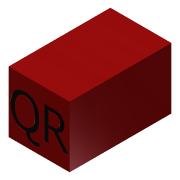
# Autodesk Inventor part: Container 2 2 2 and half color 4
Saved by Autodesk Inventor 2015 (Build 190159000, 159)
## iProperties
Created: 2015-03-07
Part Number: Container 2 2 2 and half color 4
Material: Generic
Document SubType Name: Modeling
Designer: Vukica
Density: 1 g/cm^3
Appearance: Red
Author: Vukica
Autodesk Inventor part; units mm, degrees
ref_plane "YZ Plane" through (0, 0, 0) normal (1, 0, 0) x (0, 1, 0)
ref_plane "XZ Plane" through (0, 0, 0) normal (0, 1, 0) x (-1, 0, 0)
ref_plane "XY Plane" through (0, 0, 0) normal (0, 0, 1) x (1, 0, 0)
sketch "Sketch1" plane through (0, 0, 0) normal (0, 0, 1) x (1, 0, 0)
  line L0 (0, 0) -> (38.1, 0)
  line L1 (38.1, 0) -> (38.1, 38.1)
  line L2 (38.1, 38.1) -> (0, 38.1)
  line L3 (0, 38.1) -> (0, 0)
  dimension "d0" = 38.1
  dimension "d1" = 38.1
  constraints: 8 end point, 2 parallel, 1 horizontal, 1 perpendicular
  measures "d0" distance of L1.end L2.end
  measures "d1" distance of L2.end L0.start
extrude "Extrusion1" add sketch "Sketch1" along normal blind 63.5
sketch "Sketch2" plane through (0, 0, 63.5) normal (0, 0, 1) x (1, 0, 0)
  line L0 (0.2209, 29.4428) -> (23.4184, 29.4428) construction
  line L1 (23.4184, 29.4428) -> (23.4184, 13.1304) construction
  line L2 (23.4184, 13.1304) -> (0.2209, 13.1304) construction
  line L3 (0.2209, 13.1304) -> (0.2209, 29.4428) construction
  spline S0 degree 2 poles (19.1577, 3.7217) (18.4167, 3.5406) (16.8029, 3.343) (15.996, 3.343) knots 0 0 0 1 2 2 2
  spline S1 degree 2 poles (15.996, 3.343) (13.7072, 3.343) (10.8584, 5.8953) (10.7267, 8.2666) knots 0 0 0 1 2 2 2
  spline S2 degree 2 poles (10.7267, 8.2666) (10.5455, 8.2666) (10.2327, 8.2666) (10.1009, 8.2666) knots 0 0 0 1 2 2 2
  spline S3 degree 2 poles (10.1009, 8.2666) (8.0426, 8.2666) (4.7328, 9.6662) (3.5472, 11.033) knots 0 0 0 1 2 2 2
  spline S4 degree 2 poles (3.5472, 11.033) (2.378, 12.3833) (1.1265, 16.3353) (1.1265, 18.8382) knots 0 0 0 1 2 2 2
  spline S5 degree 2 poles (1.1265, 18.8382) (1.1265, 21.407) (2.3945, 25.2932) (3.5636, 26.6764) knots 0 0 0 1 2 2 2
  spline S6 degree 2 poles (3.5636, 26.6764) (4.7492, 28.0432) (8.0591, 29.4428) (10.1009, 29.4428) knots 0 0 0 1 2 2 2
  spline S7 degree 2 poles (10.1009, 29.4428) (12.1758, 29.4428) (15.502, 27.9938) (16.6547, 26.6764) knots 0 0 0 1 2 2 2
  spline S8 degree 2 poles (16.6547, 26.6764) (17.8074, 25.3426) (19.0918, 21.3741) (19.0918, 18.8382) knots 0 0 0 1 2 2 2
  spline S9 degree 2 poles (19.0918, 18.8382) (19.0918, 14.8862) (16.0125, 9.7486) (13.3284, 8.8429) knots 0 0 0 1 2 2 2
  spline S10 degree 2 poles (13.3284, 8.8429) (13.3943, 8.0854) (13.7895, 6.8669) (14.1024, 6.5211) knots 0 0 0 1 2 2 2
  spline S11 degree 2 poles (14.1024, 6.5211) (14.4811, 6.0929) (15.5185, 5.6977) (16.4406, 5.6977) knots 0 0 0 1 2 2 2
  spline S12 degree 2 poles (16.4406, 5.6977) (16.9841, 5.6977) (18.4661, 6.0435) (18.7954, 6.1753) knots 0 0 0 1 2 2 2
  line L4 (18.7954, 6.1753) -> (19.1577, 6.1753)
  line L5 (19.1577, 6.1753) -> (19.1577, 3.7217)
  spline S13 degree 2 poles (16.276, 18.8382) (16.276, 20.8636) (15.4032, 23.9759) (14.6128, 24.9968) knots 0 0 0 1 2 2 2
  spline S14 degree 2 poles (14.6128, 24.9968) (13.806, 26.0507) (11.5335, 27.1045) (10.1174, 27.1045) knots 0 0 0 1 2 2 2
  spline S15 degree 2 poles (10.1174, 27.1045) (8.6519, 27.1045) (6.4453, 26.0836) (5.6055, 24.9968) knots 0 0 0 1 2 2 2
  spline S16 degree 2 poles (5.6055, 24.9968) (4.7986, 23.9594) (3.9424, 20.8142) (3.9424, 18.8382) knots 0 0 0 1 2 2 2
  spline S17 degree 2 poles (3.9424, 18.8382) (3.9424, 14.8368) (7.3016, 10.5719) (10.1174, 10.5719) knots 0 0 0 1 2 2 2
  spline S18 degree 2 poles (10.1174, 10.5719) (12.9332, 10.5719) (16.276, 14.8368) (16.276, 18.8382) knots 0 0 0 1 2 2 2
  line L6 (37.7816, 8.6947) -> (34.2742, 8.6947)
  line L7 (34.2742, 8.6947) -> (27.8521, 16.7799)
  line L8 (27.8521, 16.7799) -> (24.7564, 16.7799)
  line L9 (24.7564, 16.7799) -> (24.7564, 8.6947)
  line L10 (24.7564, 8.6947) -> (22.0558, 8.6947)
  line L11 (22.0558, 8.6947) -> (22.0558, 29.0147)
  line L12 (22.0558, 29.0147) -> (27.2923, 29.0147)
  spline S19 degree 2 poles (27.2923, 29.0147) (29.0377, 29.0147) (31.3925, 28.636) (32.4628, 27.9444) knots 0 0 0 1 2 2 2
  spline S20 degree 2 poles (32.4628, 27.9444) (33.5332, 27.2527) (34.7682, 25.0956) (34.7682, 23.4983) knots 0 0 0 1 2 2 2
  spline S21 degree 2 poles (34.7682, 23.4983) (34.7682, 21.2753) (32.4958, 18.2619) (30.5527, 17.5374) knots 0 0 0 1 2 2 2
  line L13 (30.5527, 17.5374) -> (37.7816, 8.6947)
  spline S22 degree 2 poles (31.9523, 23.2843) (31.9523, 24.1735) (31.3266, 25.5402) (30.6679, 25.9848) knots 0 0 0 1 2 2 2
  spline S23 degree 2 poles (30.6679, 25.9848) (30.0916, 26.3635) (28.5602, 26.6764) (27.4405, 26.6764) knots 0 0 0 1 2 2 2
  line L14 (27.4405, 26.6764) -> (24.7564, 26.6764)
  line L15 (24.7564, 26.6764) -> (24.7564, 19.0358)
  line L16 (24.7564, 19.0358) -> (27.1276, 19.0358)
  spline S24 degree 2 poles (27.1276, 19.0358) (28.2967, 19.0358) (30.1575, 19.4475) (30.7997, 20.0897) knots 0 0 0 1 2 2 2
  spline S25 degree 2 poles (30.7997, 20.0897) (31.3925, 20.6496) (31.9523, 22.2304) (31.9523, 23.2843) knots 0 0 0 1 2 2 2
  point P0 (0, 0)
  constraints: 2 other
extrude "Extrusion2" cut sketch "Sketch2" against normal blind 0.254
equation "\"d1\" = d0"
body "Solid1"
